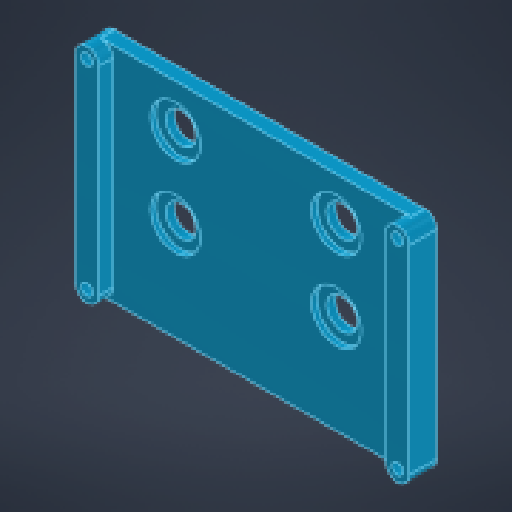
# Autodesk Inventor part: pcb
Saved by Autodesk Inventor 2024 (Build 280153000, 153)
## iProperties
Created: 2024-06-08
Part Number: pcb
Material: Generic
Document SubType Name: Modeling
Designer: markm
Density: 1 g/cm^3
Appearance: Sky Blue Dark
Author: markm
Autodesk Inventor part; units mm, degrees
ref_plane "YZ Plane" through (0, 0, 0) normal (1, 0, 0) x (0, 1, 0)
ref_plane "XZ Plane" through (0, 0, 0) normal (0, 1, 0) x (-1, 0, 0)
ref_plane "XY Plane" through (0, 0, 0) normal (0, 0, 1) x (1, 0, 0)
sketch "Sketch1" plane through (0, 0, 0) normal (0, 0, 1) x (1, 0, 0)
  line L0 (-30, -20) -> (30, -20)
  line L1 (30, -20) -> (30, 20)
  line L2 (30, 20) -> (-30, 20)
  line L3 (-30, 20) -> (-30, -20)
  line L4 (-30, -20) -> (30, 20) construction
  line L5 (30, -20) -> (-30, 20) construction
  circle A0 centre (-27.9, 17.9) radius 2.1 construction
  circle A1 centre (-27.9, 17.9) radius 1
  line L6 (0, 0) -> (-34.17, 0) construction
  line L7 (0, 33.0444) -> (0, 0) construction
  circle A2 centre (-27.9, -17.9) radius 1
  circle A3 centre (27.9, 17.9) radius 1
  circle A4 centre (27.9, -17.9) radius 1
  line L8 (-25.8, -20) -> (-25.8, 20)
  line L9 (25.8, -20) -> (25.8, 20)
  line L10 (-27.9, 17.9) -> (27.9, 17.9)
  line L11 (27.9, -17.9) -> (-27.9, -17.9)
  circle A5 centre (-14.4721, 12.2361) radius 2.75
  circle A6 centre (-14.4721, 12.2361) radius 4.5
  circle A7 centre (-14.4721, 12.2361) radius 5 construction
  circle A8 centre (-10, 10) radius 2.5 construction
  line L12 (-34.3347, 5) -> (2.7365, 5) construction
  line L13 (-14.4721, 12.2361) -> (0, 5) construction
  circle A9 centre (-14.4721, -2.2361) radius 2.75
  circle A10 centre (-14.4721, -2.2361) radius 4.5
  circle A11 centre (14.4721, 12.2361) radius 2.75
  circle A12 centre (14.4721, 12.2361) radius 4.5
  circle A13 centre (14.4721, -2.2361) radius 2.75
  circle A14 centre (14.4721, -2.2361) radius 4.5
  line L14 (-30, -10) -> (30, -10)
  arc A15 (-17.9, -10) -> (-25.8, -17.9) centre (-17.9, -17.9) ccw
  arc A16 (25.8, -17.9) -> (17.9, -10) centre (17.9, -17.9) ccw
  point P0 (-25.8, 17.9)
  point P1 (25.8, 17.9)
  point P2 (25.8, 20)
  dimension "d0" = 60
  dimension "d1" = 40
  dimension "d2" = 1.1
  dimension "d3" = 2
  dimension "d8" = 9
  dimension "d9" = 5.5
  dimension "d10" = 10
  dimension "d20" = 5
  dimension "d22" = 5
  dimension "d25" = 10
  dimension "d26" = 10
  dimension "d27" = 5
  constraints: 30 end point, 17 centre point, 14 symmetric about line, 10 point on line, 6 coincident, 5 tangent, 4 horizontal, 4 perpendicular, 4 point on circle, 3 parallel, 2 midpoint, 11 other
  measures "d0" distance of L2.end L1.end
  measures "d1" distance of L1.end L0.end
  measures "d2" distance edge to line of A1 L2
  measures "d3" diameter of A1
  measures "d8" diameter of A6
  measures "d9" diameter of A5
  measures "d10" diameter of A7
  measures "d20" diameter of A8
  measures "d22" distance of A8.centre A5.centre
  measures "d25" distance from line of A8.centre L6
  measures "d26" distance from line of A8.centre L7
  measures "d27" distance from line of A8.centre L12
extrude "Extrusion2" add sketch "Sketch1" along normal blind 2.5 contours L3 L14 L8 L0 | L3 L2 L8 L14 | L9 L14 L1 L0 | L14 L9 L2 L1
extrude "Extrusion3" add sketch "Sketch1" against normal blind 2.5 contours L3 L14 L8 L0 | L3 L2 L8 L14 | L9 L14 L1 L0 | L8 L14 A15 | L8 L10 L9 L14 | A16 L14 L9 | L2 L9 L10 L8 | L14 L9 L2 L1 | A6 | A10 | A12 | A14
extrude "Extrusion4" cut sketch "Sketch1" along normal blind 2.5 and the other way blind 1 contours A5 | A6 | A9 | A10 | A11 | A12 | A13 | A14
fillet "Fillet1" radius 2.1 8 edges at (-30, -20, 0) (-30, 20, 0) (30, -20, 0) (30, 20, 0) (-25.8, -20, 0) (-25.8, 20, 1.25) (25.8, 20, 1.25) (25.8, -20, 0)
body "Solid2"
